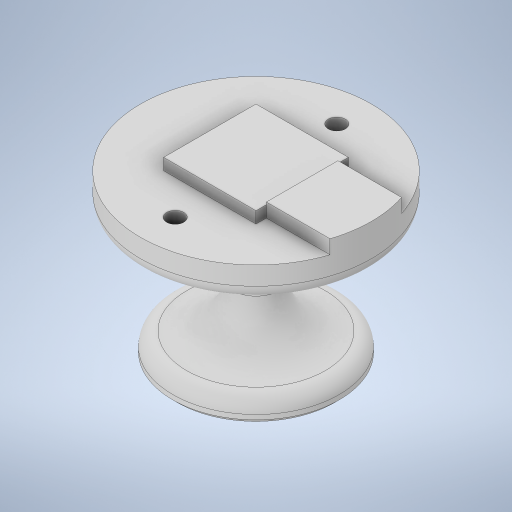
# Autodesk Inventor part: holding_socket
Saved by Autodesk Inventor 2023 (Build 270158000, 158)
## iProperties
Created: 2023-02-27
Part Number: holding_socket
Material: Generic
Document SubType Name: Modeling
Designer: maste
Density: 1 g/cm^3
Appearance: Default
Author: maste
Autodesk Inventor part; units mm, degrees
ref_plane "YZ Plane" through (0, 0, 0) normal (1, 0, 0) x (0, 1, 0)
ref_plane "XZ Plane" through (0, 0, 0) normal (0, 1, 0) x (-1, 0, 0)
ref_plane "XY Plane" through (0, 0, 0) normal (0, 0, 1) x (1, 0, 0)
sketch "Sketch2" plane through (0, 0, 0) normal (0, 0, 1) x (1, 0, 0)
  line L0 (0, 0) -> (25, 0)
  line L1 (0, 0) -> (0, 35)
  line L2 (0, 35) -> (18, 35)
  line L3 (18, 35) -> (18, 30)
  line L4 (18, 30) -> (5, 30)
  line L5 (5, 30) -> (5, 7)
  line L6 (5, 7) -> (25, 7)
  line L7 (25, 7) -> (25, 0)
  dimension "d3" = 25
  dimension "d4" = 35
  dimension "d5" = 18
  dimension "d6" = 5
  dimension "d23" = 7
  dimension "d24" = 23
  dimension "d26" = 5
  constraints: 16 end point, 6 perpendicular, 1 horizontal, 1 vertical
  measures "d3" distance of L0.start L0.end
  measures "d4" distance of L0.start L1.end
  measures "d5" distance of L1.end L2.end
  measures "d6" distance of L2.end L3.end
  measures "d23" distance of L6.end L0.end
  measures "d24" distance of L4.end L5.end
  measures "d26" distance between parallel lines of L1 L5
revolve "Revolution1" add sketch "Sketch2" angle 360 about axis through (0, 0, 0) along (0, 1, 0)
fillet "Fillet1" radius 3 3 edges at (-5, 7, 0) (-18, 30, 0) (-25, 7, 0)
chamfer "Chamfer1" distance 1 angle 45 1 edges at (-18, 35, 0)
sketch "Sketch3" plane through (0, 0, 0) normal (0, -1, 0) x (1, 0, 0)
  line L0 (0, 0) -> (0, -17.5)
  line L1 (0, 0) -> (0, 17.5)
  dimension "d14" = 17.5
  dimension "d15" = 17.5
  constraints: 4 end point, 2 coincident, 2 vertical
  measures "d14" distance of L0.start L0.end
  measures "d15" distance of L0.start L1.end
hole "Hole1" at (0, 0, 17.5) at (0, 0, -17.5) direction (0, 1, 0) diameter 3.7 depth 7 tip angle 118
fillet "Fillet2" radius 10 1 edges at (-5, 30, 0)
sketch "Sketch4" plane through (0, 7, 0) normal (0, 1, 0) x (1, 0, 0)
  circle A0 centre (0, 17.5) radius 1.85 projected
  circle A1 centre (0, -17.5) radius 1.85 projected
  circle A2 centre (0, -17.5) radius 1.85 projected
  circle A3 centre (0, -17.5) radius 1.85 projected
  point P0 (0, 0)
  constraints: 2 coincident
hole "Hole2" at (0, 7, 17.5) at (0, 7, -17.5) direction (0, -1, 0) diameter 5.75 depth 3 tip angle 118
sketch "Sketch5" plane through (0, 0, 0) normal (0, -1, 0) x (1, 0, 0)
  line L0 (-10, -10) -> (-10, 10)
  line L1 (-10, 10) -> (10, 10)
  line L2 (10, 10) -> (10, -10)
  line L3 (10, -10) -> (-10, -10)
  line L4 (-10, -10) -> (10, 10) construction
  line L5 (-10, 10) -> (10, -10) construction
  point P0 (0, 0)
  dimension "d34" = 20
  dimension "d35" = 20
  constraints: 12 end point, 2 midpoint, 2 parallel, 1 perpendicular, 1 vertical
  measures "d34" distance of L0.start L0.end
  measures "d35" distance of L0.end L1.end
extrude "Extrusion2" add sketch "Sketch5" along normal blind 2.5
chamfer "Chamfer2" distance 0.5 distance2 2 1 edges at (0, 7, 14.625) measured on face at (0, 7, 14.125)
chamfer "Chamfer3" distance 0.5 distance2 2 1 edges at (0, 7, -20.375) measured on face at (0, 7, -20.875)
sketch "Sketch7" plane through (0, 0, 0) normal (0, -1, 0) x (1, 0, 0)
  line L0 (-26, -7.75) -> (-10, -7.75)
  line L1 (-10, -7.75) -> (-10, 7.75)
  line L2 (-10, 7.75) -> (-26, 7.75)
  line L3 (-26, 7.75) -> (-26, -7.75)
  circle A0 centre (0, 0) radius 18 projected
  line L4 (-26, -7.75) -> (-10, 7.75) construction
  line L5 (-10, -7.75) -> (-26, 7.75) construction
  point P0 (-18, 0)
  dimension "d44" = 15.5
  constraints: 12 end point, 2 midpoint, 2 parallel, 1 horizontal alignment, 1 perpendicular, 1 other
  measures "d44" distance of L1.end L0.end
extrude "Extrusion3" add sketch "Sketch7" along normal blind 3 contours L3 L2 A0 L0 | A0 L2 L1 L0 picked at (-12.6667, 0)
sketch "Sketch8" plane through (-10, 0, 10) normal (0, -1, 0) x (1, 0, 0)
  arc A0 (-13.7684, -17.75) -> (-13.7684, -2.25) centre (10, -10) ccw projected
  line L0 (-12.5073, 0.8822) -> (-22.2437, 0.8822)
  line L1 (-22.2437, 0.8822) -> (-22.2437, -21.0128)
  line L2 (-22.2437, -21.0128) -> (-12.5073, -21.0128)
  line L3 (-12.5073, -21.0128) -> (-12.4075, -21.0862)
  arc A1 (-12.5073, 0.8822) -> (-12.4075, -21.0862) centre (10, -10) ccw
  point P0 (-13.7684, -2.25)
  constraints: 8 end point, 4 point on circle, 1 centre point, 1 concentric, 1 horizontal, 1 parallel, 1 perpendicular
extrude "Extrusion4" cut sketch "Sketch8" along normal blind 7.25 contours A0 L3 L2 L1 L0 A1
chamfer "Chamfer4" [suppressed]
fillet "Fillet3" [suppressed]
body "Solid2"
